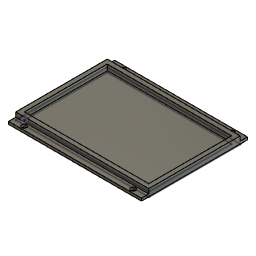
BreadBoard Mount v6 (Autodesk Fusion 360 design; units mm, degrees)
Autodesk Fusion 360 part; units mm, degrees
sketch "Sketch1" plane through (0, 0, 0) normal (0, 1, 0) x (1, 0, 0)
  line L0 (0, 0) -> (87, 0)
  line L1 (87, 0) -> (87, 58)
  line L2 (87, 58) -> (0, 58)
  line L3 (0, 58) -> (0, 0)
  line L4 (-3, 61) -> (90, 61)
  line L5 (90, 61) -> (90, -3)
  line L6 (90, -3) -> (-3, -3)
  line L7 (-3, -3) -> (-3, 61)
  dimension "d1" = 87
  dimension "d2" = 58
  dimension "d3" = 3
  dimension "d4" = 3
  dimension "d5" = 3
  dimension "d6" = 3
  constraint horizontal L0
  constraint vertical L1
  constraint horizontal L2
  constraint vertical L3
  constraint coincident L0.start L3.end
  constraint horizontal L4
  constraint vertical L5
  constraint horizontal L6
  constraint vertical L7
  measures "d1" distance of L0.start L0.end
  measures "d2" distance of L0.start L2.end
  measures "d3" distance of L1 L5
  measures "d4" distance of L0 L6
  measures "d5" distance of L3 L7
  measures "d6" distance of L2 L4
extrude "Extrude1" add sketch "Sketch1" along normal blind 5
extrude "Extrude2" add sketch "Sketch1" along normal blind 1 contours L0 L1 L2 L3
sketch "Sketch2" plane through (0, 0, 0) normal (0, 1, 0) x (1, 0, 0)
  line L0 (90, -3) -> (-3, -3)
  line L1 (-3, -3) -> (-3, 61)
  line L2 (-3, 61) -> (90, 61)
  line L3 (90, 61) -> (90, -3)
  circle A0 centre (81.6, 63.54) radius 1.75
  circle A1 centre (5.4, 63.54) radius 1.75
  line L4 (-3, -3) -> (-3, 61)
  line L5 (-3, 61) -> (90, 61)
  circle A2 centre (81.6, -5.54) radius 1.75
  circle A3 centre (5.4, -5.54) radius 1.75
  line L6 (90, -3) -> (-3, -3)
  line L7 (-3, 66.08) -> (90, 66.08)
  line L8 (90, 66.08) -> (90, -8.08)
  line L9 (90, -8.08) -> (-3, -8.08)
  line L10 (-3, -8.08) -> (-3, 66.08)
  dimension "d11" = 3.5
  dimension "d12" = 3.5
  dimension "d13" = 76.2
  dimension "d14" = 8.4
  dimension "d15" = 2.54
  dimension "d16" = 3.5
  dimension "d17" = 3.5
  dimension "d18" = 2.54
  dimension "d19" = 2.54
  dimension "d21" = 2.54
  dimension "d22" = 2.54
  constraint horizontal L7
  constraint vertical L8
  constraint horizontal L9
  constraint vertical L10
  measures "d11" diameter of A0
  measures "d12" diameter of A1
  measures "d13" distance of A0.centre A1.centre
  measures "d14" distance of A1.centre L4
  measures "d15" distance of A0.centre L5
  measures "d16" diameter of A2
  measures "d17" diameter of A3
  measures "d18" distance of A3.centre L6
  measures "d19" distance of A2.centre L6
  measures "d21" distance of A3.centre L9
  measures "d22" distance of A0.centre L7
extrude "Extrude3" add sketch "Sketch2" along normal blind 1.778 contours L0 L6 L8 L9 L10 | L2 L5 L7 L8 L10
equation "d4 = d3"
equation "d5 = d4"
